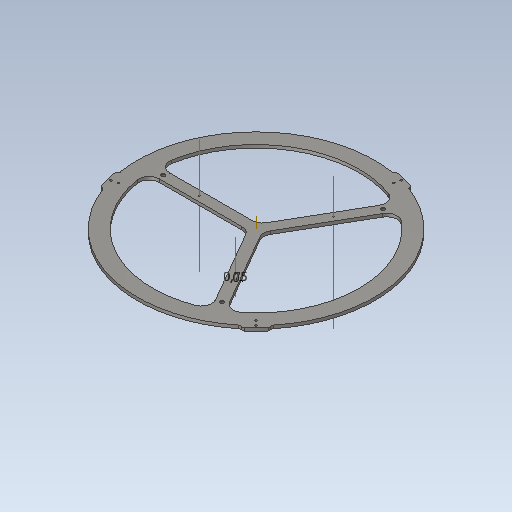
# Autodesk Inventor part: PrimaryMirror
Saved by Autodesk Inventor 2020 (Build 240168000, 168)
## iProperties
Created: 2019-04-25
Part Number: PrimaryMirror
Material: Stal nierdzewna
Document SubType Name: Modeling
Designer: barto
Density: 8 g/cm^3
Appearance: Częściowo polerowana
Author: barto
Autodesk Inventor part; units mm, degrees
ref_plane "YZ Plane" through (0, 0, 0) normal (1, 0, 0) x (0, 1, 0)
ref_plane "XZ Plane" through (0, 0, 0) normal (0, 1, 0) x (-1, 0, 0)
sketch "Szkic1" plane through (0, 0, 0) normal (0, 1, 0) x (-1, 0, 0)
  circle A0 centre (0, 0) radius 115
  circle A1 centre (0, 0) radius 94.4395
  dimension "d52" = 230
  constraints: 2 centre point, 2 coincident
  measures "d52" diameter of A0
extrude "Wyciągnięcie proste1" add sketch "Szkic1" along normal blind 3 contours A0 | A1
sketch "Szkic2" plane through (0, 3, 0) normal (0, 1, 0) x (1, 0, 0)
  line L0 (-2.8868, 5) -> (-99.8749, 5)
  line L1 (-99.8749, -5) -> (-2.8868, -5)
  line L2 (-2.8868, -5) -> (45.6073, -88.9942)
  line L3 (54.2676, -83.9942) -> (5.7735, 0)
  line L4 (5.7735, 0) -> (54.2676, 83.9942)
  line L5 (45.6073, 88.9942) -> (-2.8868, 5)
  arc A0 (45.6073, 88.9942) -> (-99.8749, 5) centre (0, 0) ccw
  arc A1 (-99.8749, -5) -> (45.6073, -88.9942) centre (0, 0) ccw
  arc A2 (54.2676, -83.9942) -> (54.2676, 83.9942) centre (0, 0) ccw
  arc A3 (45.6073, 88.9942) -> (-99.8749, 5) centre (0, 0) ccw
  line L6 (-99.8749, 5) -> (-2.8868, 5)
  line L7 (45.6073, 88.9942) -> (-2.8868, 5)
  dimension "d12" = 10
  dimension "d13" = 5
  dimension "d20" = 360
  dimension "d22" = 100
  constraints: 16 end point, 8 point on circle, 4 centre point, 3 equal length, 2 coincident, 1 concentric, 1 horizontal, 1 point on line, 19 other
  measures "d12" distance between parallel lines of L1 L0
  measures "d13" distance from line of L0 point (0, 0)
  measures "d22" radius of A0
extrude "Wyciągnięcie proste2" cut sketch "Szkic2" against normal blind 3 contours L0 A0 L5
pattern_circular "Szyk kołowy1" count 3 over 360 about axis through (0, 3, 0) along (0, 1, 0) of "Wyciągnięcie proste2"
sketch "Szkic3" plane through (0, 3, 0) normal (0, 1, 0) x (1, 0, 0)
  line L0 (5.7735, 0) -> (54.2676, 83.9942) projected
  circle A0 centre (0, 0) radius 90
  point P0 (45, 77.9423)
  point P1 (-90, 0)
  point P2 (45, -77.9423)
  dimension "d54" = 180
  dimension "d83" = 360
  constraints: 1 centre point, 1 coincident, 4 other
  measures "d54" diameter of A0
sketch "Szkic4" plane through (0, 0, 0) normal (0, -1, 0) x (1, 0, 0)
  line L0 (5.7735, 0) -> (54.2676, 83.9942) projected
  circle A0 centre (27.5, 47.6314) radius 0.75
  circle A1 centre (-55, 0) radius 0.75
  circle A2 centre (27.5, -47.6314) radius 0.75
  point P0 (0, 0)
  dimension "d44" = 5
  dimension "d45" = 1.5
  dimension "d48" = 360
  constraints: 3 centre point, 3 coincident, 10 other
  measures "d44" distance from line of L0 point (27.5, 47.631)
  measures "d45" diameter of A0
extrude "Wyciągnięcie proste4" cut sketch "Szkic4" against normal blind 10
fillet "Zaokrąglenie1" radius 10 9 edges at (5.7735, 1.5, 0) (-2.8868, 1.5, -5) (-2.8868, 1.5, 5) (-99.8749, 1.5, 5) (-99.8749, 1.5, -5) (54.2676, 1.5, 83.9942) (45.6073, 1.5, 88.9942) (45.6073, 1.5, -88.9942) (54.2676, 1.5, -83.9942)
sketch "Szkic5" plane through (0, 0, 0) normal (0, -1, 0) x (1, 0, 0)
  circle A0 centre (27.5, 47.6314) radius 0.75 projected
  line L0 (28.25, 47.6314) -> (28.25, 50.8241)
  point P0 (0, 0)
  dimension "d56" = 0
  dimension "d59" = 0.75
  constraints: 2 end point, 1 vertical
  measures "d56" vertical distance of A0.centre L0.start
  measures "d59" distance of A0.centre L0.start
ref_plane "Płaszczyzna konstrukcyjna1" through (28.25, 0, 47.6314) normal (0, 0, 1) x (1, 0, 0)
sketch "Szkic7" plane through (0, 0, 0) normal (0, -1, 0) x (1, 0, 0)
  point P0 (0, 0)
sketch "Szkic8" plane through (28.25, 0, 47.6314) normal (0, 0, 1) x (1, 0, 0)
  line L0 (0, 0) -> (-1.5, 0) projected
  line L1 (-0.75, 1.5) -> (-0.75, 0)
  line L2 (-0.75, 0) -> (1.8481, 0)
  line L3 (1.8481, 0) -> (-0.75, 1.5)
  line L4 (-0.75, -0.6) -> (-0.75, 3.6) projected
  point P0 (-28.25, 0)
  dimension "d61" = 1.5
  dimension "d62" = 60
  constraints: 6 end point, 1 horizontal, 1 midpoint, 1 vertical
  measures "d61" distance of L1.end L1.start
  measures "d62" angle of L1 L3
revolve "Obrót1" cut sketch "Szkic8" angle 360 about axis through (27.5, 0, 47.6314) along (0, 1, 0)
pattern_circular "Szyk kołowy2" count 3 over 360 about axis through (0, 3, 0) along (0, 1, 0) of "Obrót1"
sketch "Szkic10" plane through (0, 0, 0) normal (0, -1, 0) x (1, 0, 0)
  line L0 (0, 0) -> (-84.2181, 0)
  circle A0 centre (0, 0) radius 115 projected
  line L1 (0, 0) -> (-150.0694, 40.211)
  circle A1 centre (0, 0) radius 115
  circle A2 centre (0, 0) radius 109
  point P0 (29.2466, -109.1496)
  point P1 (27.6936, -103.3541)
  point P2 (79.9031, 79.9031)
  point P3 (75.6604, 75.6604)
  point P4 (-111.0815, 29.7642)
  point P5 (-105.2859, 28.2113)
  point P6 (28.2113, -105.2859)
  point P7 (29.7642, -111.0815)
  point P8 (77.0746, 77.0746)
  point P9 (81.3173, 81.3173)
  dimension "d72" = 230
  dimension "d73" = 218
  dimension "d71" = 15
  dimension "d111" = 360
  constraints: 4 end point, 2 coincident, 2 point on line, 1 horizontal, 13 other
  measures "d71" angle of L0 L1
hole "Otwór1" at (45, 3, -77.9423) at (-90, 3, 0) at (45, 3, 77.9423) direction (0, -1, 0) diameter 3.242 end through all thread size "M4x0.7" class "6H" standard "ISO Metric profile"
chamfer "Faza1" distance 0.4 angle 45 3 edges at (45, 3, -79.5633) (-90, 3, -1.621) (45, 3, 76.3213)
sketch "Szkic11" plane through (0, 0, 0) normal (0, -1, 0) x (1, 0, 0)
  arc A0 (-115, 0) -> (-115, 0) centre (0, 0) ccw projected
  arc A1 (-115, 0) -> (-115, 0) centre (0, 0) ccw projected
  circle A2 centre (-90, 0) radius 1.621 projected
  line L0 (0, 0) -> (-90, 0)
  line L1 (-108.0647, 39.3323) -> (-110.4139, 40.1874)
  line L2 (-113.2529, 19.9695) -> (-115.7149, 20.4037)
  arc A3 (-110.4139, 40.1874) -> (-115.7149, 20.4037) centre (0, 0) ccw
  line L3 (-113.2529, 19.9695) -> (-108.0647, 39.3323)
  line L4 (-110.4139, 40.1874) -> (-115.7149, 20.4037)
  dimension "d120" = 20
  dimension "d121" = 10
  dimension "d122" = 235
  constraints: 10 end point, 4 point on circle, 1 centre point, 1 coincident, 1 horizontal
  measures "d120" angle of L1 L0
  measures "d121" angle of L2 L0
  measures "d122" diameter of A3
extrude "Wyciągnięcie proste6" add sketch "Szkic11" against normal blind 3 contours L3 A0 | A0 L2 L4 L1 | L4 A3 picked at (-110.4955, 30.7614)
pattern_circular "Szyk kołowy4" count 3 over 360 about axis through (0, 3, 0) along (0, 1, 0) of "Wyciągnięcie proste6"
hole "Otwór4" at (-111.0815, 0, 29.7642) at (-105.2859, 0, 28.2113) at (81.3173, 0, 81.3173) at (77.0746, 0, 77.0746) at (28.2113, 0, -105.2859) at (29.7642, 0, -111.0815) direction (0, 1, 0) diameter 2.013 depth 7.6 tip angle 118 thread size "M2.5x0.45" class "6H" standard "ISO Metric profile"
fillet "Zaokrąglenie2" radius 2 12 edges at (-113.2529, 1.5, 19.9695) (-115.7149, 1.5, 20.4037) (-108.0647, 1.5, 39.3323) (-110.4139, 1.5, 40.1874) (20.4037, 1.5, -115.7149) (19.9695, 1.5, -113.2529) (40.1874, 1.5, -110.4139) (39.3323, 1.5, -108.0647) (90.0102, 1.5, 75.5275) (88.0951, 1.5, 73.9206) (75.5275, 1.5, 90.0102) (73.9206, 1.5, 88.0951)
